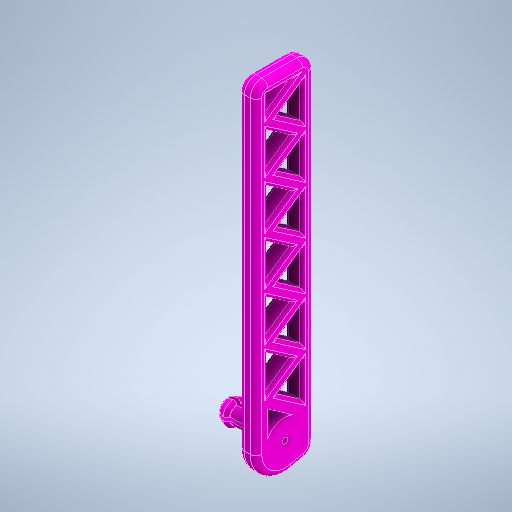
# Autodesk Inventor part: Reverse Lockout
Saved by Autodesk Inventor 2025.2 (Build 292293000, 293)
## iProperties
Created: 2025-02-09
Part Number: Reverse Lockout
Material: Generic
Document SubType Name: Modeling
Designer: eason
Density: 1 g/cm^3
Appearance: Magenta
Author: eason
Autodesk Inventor part; units mm, degrees
ref_plane "YZ Plane" through (0, 0, 0) normal (1, 0, 0) x (0, 1, 0)
ref_plane "XZ Plane" through (0, 0, 0) normal (0, 1, 0) x (-1, 0, 0)
sketch "Sketch3" plane through (0, 0, 0) normal (0, 0, 1) x (1, 0, 0)
  line L0 (0, 0) -> (3, 0)
  line L1 (3, 0) -> (3, 60)
  line L2 (3, 60) -> (0, 60)
  line L3 (0, 60) -> (0, 0)
  dimension "d12" = 3
  dimension "d13" = 60
  constraints: 8 end point, 2 parallel, 1 horizontal, 1 perpendicular
  measures "d12" distance between parallel lines of L3 L1
  measures "d13" distance between parallel lines of L0 L2
extrude "Extrusion3" add sketch "Sketch3" along normal blind 10
sketch "Sketch4" plane through (3, 0, 0) normal (1, 0, 0) x (0, 0, -1)
  circle A0 centre (-5, 5) radius 5
  line L0 (0, 0) -> (-10, 0) projected
  line L1 (0, 0) -> (0, 60) projected
  line L2 (0, 0) -> (0, 60) projected
  line L3 (0, 60) -> (-10, 60) projected
  line L4 (-10, 0) -> (-10, 60) projected
  line L5 (0, 0) -> (-10, 0) projected
  line L6 (-3.9024, 0.122) -> (0, 1)
  point P0 (-10, 5)
  point P1 (-10, 0)
  point P2 (-5, 0)
  dimension "d16" = 10
  dimension "d20" = 1
  constraints: 2 end point, 1 horizontal, 1 point on line, 1 vertical, 4 other
  measures "d20" distance from line of L0 L6.end
extrude "Extrusion4" cut sketch "Sketch4" against normal through all contours L6 L1 L0 A0 | L0 L4 A0
sketch "Sketch7" plane through (0, 60, 0) normal (-1, 0, 0) x (0, 0, 1)
  line L0 (2, -2) -> (8, -2)
  line L1 (8, -2) -> (8, -53.1972)
  line L2 (2, -53.1972) -> (2, -2)
  line L3 (0, 0) -> (0, -59) projected
  line L4 (10, 0) -> (10, -55) projected
  line L5 (0, 0) -> (10, 0) projected
  line L6 (2, -10.2879) -> (8, -10.2879) construction
  line L7 (2, -2) -> (8, -6.1439) construction
  line L8 (8, -6.1439) -> (2, -10.2879) construction
  line L9 (3.7597, -2) -> (8, -4.9286)
  line L10 (2, -3.2153) -> (6.2403, -6.1439)
  line L11 (6.2403, -6.1439) -> (2, -9.0725)
  line L12 (3.7597, -10.2879) -> (8, -7.3592)
  line L13 (2, -18.5757) -> (8, -18.5757) construction
  line L14 (3.7597, -18.5757) -> (8, -15.6471)
  line L15 (2, -17.3604) -> (6.2403, -14.4318)
  line L16 (6.2403, -14.4318) -> (2, -11.5032)
  line L17 (3.7597, -10.2879) -> (8, -13.2165)
  line L18 (2, -26.8636) -> (8, -26.8636) construction
  line L19 (3.7597, -18.5757) -> (8, -21.5043)
  line L20 (2, -19.791) -> (6.2403, -22.7196)
  line L21 (6.2403, -22.7196) -> (2, -25.6483)
  line L22 (3.7597, -26.8636) -> (8, -23.935)
  line L23 (2, -35.1514) -> (8, -35.1514) construction
  line L24 (3.7597, -26.8636) -> (8, -29.7922)
  line L25 (6.2403, -31.0075) -> (2, -28.0789)
  line L26 (2, -33.9361) -> (6.2403, -31.0075)
  line L27 (3.7597, -35.1514) -> (8, -32.2228)
  line L28 (2, -43.4393) -> (8, -43.4393) construction
  line L29 (3.7597, -35.1514) -> (8, -38.08)
  line L30 (2, -36.3668) -> (6.2403, -39.2954)
  line L31 (6.2403, -39.2954) -> (2, -42.224)
  line L32 (3.7597, -43.4393) -> (8, -40.5107)
  line L33 (2, -51.7271) -> (8, -51.7271) construction
  line L34 (3.7597, -43.4393) -> (8, -46.3679)
  line L35 (6.2403, -47.5832) -> (2, -44.6546)
  line L36 (2, -50.5118) -> (6.2403, -47.5832)
  line L37 (3.7597, -51.7271) -> (8, -48.7985)
  arc A0 (8, -53.1972) -> (2, -53.1972) centre (5, -55) ccw
  arc A1 (3.9024, -59.878) -> (10, -55) centre (5, -55) ccw projected
  point P0 (0, -60)
  point P1 (2, -11.5032)
  point P2 (2, -17.3604)
  point P3 (8, -13.2165)
  point P4 (8, -15.6471)
  point P5 (2, -19.791)
  point P6 (2, -25.6483)
  point P7 (2, -28.0789)
  point P8 (2, -33.9361)
  point P9 (8, -29.7922)
  point P10 (8, -23.935)
  point P11 (2, -36.3668)
  point P12 (2, -42.224)
  point P13 (2, -44.6546)
  point P14 (2, -50.5118)
  point P15 (8, -46.3679)
  point P16 (8, -48.7985)
  dimension "d45" = 2
  dimension "d46" = 2
  dimension "d47" = 2
  dimension "d51" = 1
  dimension "d52" = 2
  dimension "d53" = 2
  dimension "d58" = 3.5
  constraints: 70 end point, 40 symmetric about line, 14 point on line, 4 parallel, 3 equal length, 3 point on circle, 2 perpendicular, 1 centre point, 1 concentric, 1 horizontal
  measures "d45" distance between parallel lines of L3 L2
  measures "d46" distance between parallel lines of L4 L1
  measures "d47" distance between parallel lines of L5 L0
  measures "d51" distance between parallel lines of L7 L9
  measures "d52" distance between parallel lines of L10 L9
  measures "d53" distance between parallel lines of L12 L11
  measures "d58" radius of A0
extrude "Extrusion7" cut sketch "Sketch7" against normal through all contours L0 L1 L9 | L10 L11 L2 | L1 L17 L12 | L16 L15 L2 | L1 L19 L14 | L20 L21 L2 | L1 L24 L22 | L25 L26 L2 | L1 L29 L27 | L30 L31 L2 | L1 L34 L32 | L35 L36 L2 | L1 A0 L37
fillet "Fillet2" radius 2 3 edges at (1.5, 60, 0) (1.5, 60, 10) (1.5, 1, 0)
fillet "Fillet3" radius 1 16 edges at (3, 59.4142, 0.5858) (3, 60, 5) (3, 59.4142, 9.4142) (3, 31.5, 10) (3, 1.0957, 8.1235) (3, 0.3854, 2.7317) (3, 1.3506, 0.4383) (3, 30.3, 0) (0, 1.3506, 0.4383) (0, 0.3854, 2.7317) (0, 1.0957, 8.1235) (0, 31.5, 10) (0, 59.4142, 9.4142) (0, 60, 5) (0, 59.4142, 0.5858) (0, 30.3, 0)
fillet "Fillet4" radius 0.5 72 edges at (3, 53.8561, 2) (3, 52.3918, 4.1202) (3, 55.3204, 4.1202) (3, 51.1764, 5.8798) (3, 48.2478, 5.8798) (3, 49.7121, 8) (3, 56.5357, 5.8798) (3, 58, 5.8798) (3, 56.5357, 8) (3, 47.0325, 4.1202) (3, 45.5682, 2) (3, 44.1039, 4.1202) (3, 42.8886, 5.8798) (3, 41.4243, 8) (3, 39.96, 5.8798) (3, 38.7447, 4.1202) (3, 37.2804, 2) (3, 35.8161, 4.1202) (3, 34.6007, 5.8798) (3, 33.1364, 8) (3, 31.6721, 5.8798) (3, 30.4568, 4.1202) (3, 28.9925, 2) (3, 27.5282, 4.1202) (3, 26.3129, 5.8798) (3, 24.8486, 8) (3, 23.3843, 5.8798) (3, 22.1689, 4.1202) (3, 20.7046, 2) (3, 19.2403, 4.1202) (3, 18.025, 5.8798) (3, 16.5607, 8) (3, 15.0964, 5.8798) (3, 13.8811, 4.1202) (3, 12.4168, 2) (3, 10.9525, 4.1202) (0, 10.9525, 4.1202) (0, 12.4168, 2) (0, 13.8811, 4.1202) (0, 15.0964, 5.8798) (0, 18.025, 5.8798) (0, 16.5607, 8) (0, 19.2403, 4.1202) (0, 20.7046, 2) (0, 22.1689, 4.1202) (0, 23.3843, 5.8798) (0, 24.8486, 8) (0, 26.3129, 5.8798) (0, 27.5282, 4.1202) (0, 28.9925, 2) (0, 30.4568, 4.1202) (0, 31.6721, 5.8798) (0, 33.1364, 8) (0, 34.6007, 5.8798) (0, 35.8161, 4.1202) (0, 37.2804, 2) (0, 38.7447, 4.1202) (0, 39.96, 5.8798) (0, 41.4243, 8) (0, 42.8886, 5.8798) (0, 44.1039, 4.1202) (0, 45.5682, 2) (0, 47.0325, 4.1202) (0, 48.2478, 5.8798) (0, 49.7121, 8) (0, 51.1764, 5.8798) (0, 52.3918, 4.1202) (0, 53.8561, 2) (0, 55.3204, 4.1202) (0, 56.5357, 5.8798) (0, 56.5357, 8) (0, 58, 5.8798)
sketch "Sketch8" plane through (0, 2.6, 1) normal (-1, 0, 0) x (0, 0, 1)
  circle A0 centre (4, 2.4) radius 1.5
  arc A1 (7, 4.2028) -> (2.7597, 5.6729) centre (4, 2.4) ccw projected
  point P0 (-1, -2.6)
  dimension "d59" = 3
  constraints: 1 centre point, 1 concentric
  measures "d59" diameter of A0
extrude "Extrusion8" add sketch "Sketch8" along normal blind 7
ref_plane "Work Plane1" through (0, 5, 5) normal (0, 0, -1) x (-1, 0, 0)
sketch "Sketch9" plane through (0, 5, 5) normal (0, 0, -1) x (-1, 0, 0)
  line L0 (0, 1.5) -> (7, 1.5) projected
  line L1 (7, -1.5) -> (7, 1.5) projected
  line L2 (7, 1.5) -> (5, 2.3)
  line L3 (5, 2.3) -> (5, 1.5)
  line L4 (7, 0) -> (0, 0)
  line L5 (0, -2.4) -> (0, 53) projected
  point P0 (0, -5)
  dimension "d62" = 2
  dimension "d63" = 0.8
  constraints: 6 end point, 2 point on line, 1 horizontal, 1 midpoint, 1 perpendicular
  measures "d62" distance between parallel lines of L1 L3
  measures "d63" distance of L2.end L3.end
revolve "Revolution1" add sketch "Sketch9" angle 360 about axis through (-7, 5, 5) along (1, 0, 0) contours L3 L2 L0
sketch "Sketch10" plane through (-7, 5, 5) normal (-1, 0, 0) x (0, 0, 1)
  circle A0 centre (0, 0) radius 0.5
  circle A1 centre (0, 0) radius 1.5 projected
  point P0 (-5, -5)
  dimension "d65" = 1
  constraints: 1 centre point
  measures "d65" radial gap between concentric circles of A0 A1
extrude "Extrusion9" cut sketch "Sketch10" against normal through all contours A0
sketch "Sketch11" plane through (-7, 5, 5) normal (-1, 0, 0) x (0, 0, 1)
  circle A0 centre (0, 0) radius 0.5 projected
  line L0 (-0.4, -0.3) -> (-2.2804, -0.3)
  circle A1 centre (0, 0) radius 2.3 projected
  line L1 (-2.2804, 0.3) -> (-0.4, 0.3)
  line L2 (0.3, -0.4) -> (0.3, -2.2804)
  line L3 (-0.3, -2.2804) -> (-0.3, -0.4)
  line L4 (0.4, 0.3) -> (2.2804, 0.3)
  line L5 (2.2804, -0.3) -> (0.4, -0.3)
  line L6 (-0.3, 0.4) -> (-0.3, 2.2804)
  line L7 (0.3, 2.2804) -> (0.3, 0.4)
  point P0 (-5, -5)
  point P1 (-0.3, -0.4)
  point P2 (-0.3, -2.2804)
  point P3 (0.3, -2.2804)
  point P4 (0.3, -0.4)
  point P5 (0.4, -0.3)
  point P6 (2.2804, 0.3)
  point P7 (0.4, 0.3)
  point P8 (0.3, 0.4)
  point P9 (0.3, 2.2804)
  point P10 (-0.3, 2.2804)
  point P11 (-0.3, 0.4)
  dimension "d68" = 0.6
  dimension "d69" = 0.3
  dimension "d72" = 360
  constraints: 16 end point, 4 point on circle, 2 horizontal, 25 other
  measures "d68" distance between parallel lines of L1 L0
  measures "d69" distance from line of L0 A0.centre
extrude "Extrusion10" cut sketch "Sketch11" against normal up to surface (7 mm away) contours A0 L4 A1 L5 | A0 L6 A1 L7 | L2 A1 L3 A0 | A0 L0 A1 L1
fillet "Fillet5" radius 0.5 8 edges at (-5, 3.3737, 3.3737) (-5, 6.6263, 3.3737) (-5, 6.6263, 6.6263) (-5, 3.3737, 6.6263) (-7, 3.9393, 3.9393) (-7, 6.0607, 3.9393) (-7, 6.0607, 6.0607) (-7, 3.9393, 6.0607)
equation "\"d45\" = b"
equation "\"d46\" = b"
equation "\"d47\" = b"
equation "\"d51\" = 0.5 * b"
equation "\"d52\" = b"
equation "\"d53\" = b"
equation "\"b\" = 2"
body "Solid2"
